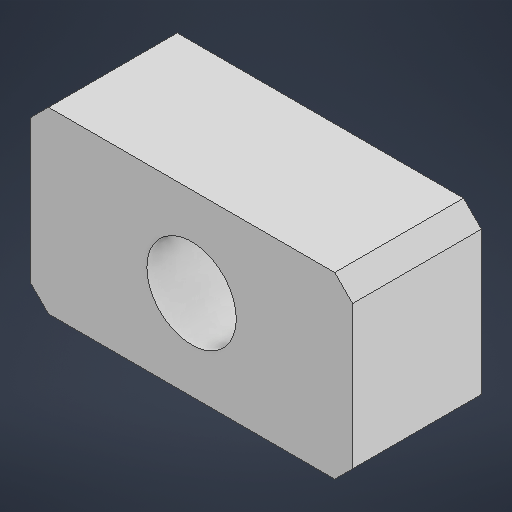
# Autodesk Inventor part: Slide
Saved by Autodesk Inventor 2025.4 (Build 294407000, 407)
## iProperties
Created: 2026-05-29
Part Number: Slide
Material: Generic
Document SubType Name: Modeling
Designer: VuQuan
Density: 1 g/cm^3
Appearance: Default
Author: VuQuan
Autodesk Inventor part; units mm, degrees
ref_plane "YZ Plane" through (0, 0, 0) normal (1, 0, 0) x (0, 1, 0)
ref_plane "XZ Plane" through (0, 0, 0) normal (0, 1, 0) x (-1, 0, 0)
ref_plane "XY Plane" through (0, 0, 0) normal (0, 0, 1) x (1, 0, 0)
sketch "Sketch1" plane through (0, 0, 0) normal (0, 0, 1) x (1, 0, 0)
  circle A0 centre (0, 0) radius 2.5
  line L0 (-8, 5) -> (8, 5)
  line L1 (9, 4) -> (9, -4)
  line L2 (8, -5) -> (-8, -5)
  line L3 (-9, -4) -> (-9, 4)
  line L4 (-8, 5) -> (-9, 4)
  line L5 (-9, -4) -> (-8, -5)
  line L6 (8, -5) -> (9, -4)
  line L7 (9, 4) -> (8, 5)
  point P0 (-9, 5)
  point P1 (9, -5)
  point P2 (9, 5)
  point P3 (-9, -5)
  point P4 (0, 5)
  point P5 (9, 0)
  dimension "d0" = 5
  dimension "d1" = 1
  dimension "d2" = 1
  dimension "d3" = 1
  dimension "d4" = 1
  dimension "d5" = 1
  dimension "d6" = 1
  dimension "d7" = 1
  dimension "d8" = 1
  dimension "d9" = 18
  dimension "d10" = 10
  constraints: 16 end point, 8 point on line, 2 midpoint, 2 parallel, 1 centre point, 1 coincident, 1 horizontal, 1 horizontal alignment, 1 perpendicular, 1 vertical alignment
  measures "d0" diameter of A0
  measures "d1" distance of L0.start point (-9, 5)
  measures "d2" distance of L3.end point (-9, 5)
  measures "d3" distance of L3.start point (-9, -5)
  measures "d4" distance of L2.end point (-9, -5)
  measures "d5" distance of L2.start point (9, -5)
  measures "d6" distance of L1.end point (9, -5)
  measures "d7" distance of L1.start point (9, 5)
  measures "d8" distance of L0.end point (9, 5)
  measures "d9" distance between parallel lines of L1 L3
  measures "d10" distance between parallel lines of L0 L2
extrude "Extrusion1" add sketch "Sketch1" along normal blind 7.2
equation "\"d2\" = d1"
equation "\"d3\" = d1"
equation "\"d4\" = d3"
equation "\"d5\" = d1"
equation "\"d6\" = d5"
equation "\"d7\" = d1"
equation "\"d8\" = d7"
body "Solid1"
